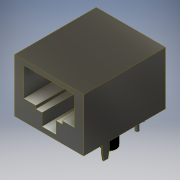
# Autodesk Inventor part: RJE051AA1310
Saved by Autodesk Inventor 2016 (Build 200138000, 138)
## iProperties
Created: 2016-08-10
Part Number: RJE051AA1310
Material: Generic
Document SubType Name: Modeling
Designer: jfixelle
Density: 1 g/cm^3
Appearance: Silver
Author: jfixelle
Autodesk Inventor part; units mm, degrees
ref_plane "YZ Plane" through (0, 0, 0) normal (1, 0, 0) x (0, 1, 0)
ref_plane "XZ Plane" through (0, 0, 0) normal (0, 1, 0) x (-1, 0, 0)
ref_plane "XY Plane" through (0, 0, 0) normal (0, 0, 1) x (1, 0, 0)
sketch "Sketch1" plane through (0, 0, 0) normal (0, 1, 0) x (-1, 0, 0)
  line L0 (7.95, 14.5) -> (-7.95, 14.5)
  line L1 (-7.95, 14.5) -> (-7.95, -4.3)
  line L2 (-7.95, -4.3) -> (7.95, -4.3)
  line L3 (7.95, -4.3) -> (7.95, 14.5)
  point P0 (0, 0)
  dimension "d0" = 18.8
  dimension "d1" = 15.9
  dimension "d2" = 7.95
  dimension "d5" = 14.5
  constraints: 8 end point, 2 parallel, 1 horizontal, 1 perpendicular
  measures "d0" distance of L2.end L0.start
  measures "d1" distance of L1.end L2.end
  measures "d2" distance from line of point (0, 0) L3
  measures "d5" distance from line of point (0, 0) L0
extrude "Extrusion1" add sketch "Sketch1" along normal blind 12.25
sketch "Sketch2" plane through (-7.95, 0, 14.5) normal (0, 0, 1) x (1, 0, 0)
  line L0 (2.12, 11.155) -> (13.78, 11.155)
  line L1 (13.78, 11.155) -> (13.78, 4.555)
  line L2 (13.78, 4.555) -> (2.12, 4.555)
  line L3 (2.12, 4.555) -> (2.12, 11.155)
  line L4 (4.9, 4.555) -> (11, 4.555)
  line L5 (11, 4.555) -> (11, 3.865)
  line L6 (11, 3.865) -> (4.9, 3.865)
  line L7 (4.9, 3.865) -> (4.9, 4.555)
  line L8 (6.325, 3.865) -> (9.575, 3.865)
  line L9 (9.575, 3.865) -> (9.575, 1.095)
  line L10 (9.575, 1.095) -> (6.325, 1.095)
  line L11 (6.325, 1.095) -> (6.325, 3.865)
  line L12 (0, 12.25) -> (15.9, 12.25) projected
  point P0 (7.95, 0)
  dimension "d6" = 11.66
  dimension "d7" = 5.83
  dimension "d8" = 6.1
  dimension "d9" = 3.05
  dimension "d10" = 3.25
  dimension "d11" = 1.625
  dimension "d12" = 7.29
  dimension "d13" = 2.77
  dimension "d14" = 6.6
  dimension "d16" = 1.095
  constraints: 24 end point, 6 parallel, 3 horizontal, 3 perpendicular, 2 point on line
  measures "d6" distance of L0.start L0.end
  measures "d7" distance from line of point (7.95, 0) L1
  measures "d8" distance of L5.end L6.end
  measures "d9" distance from line of point (7.95, 0) L5
  measures "d10" distance of L9.end L10.end
  measures "d11" distance from line of point (7.95, 0) L9
  measures "d12" distance between parallel lines of L6 L0
  measures "d13" distance between parallel lines of L10 L6
  measures "d14" distance between parallel lines of L2 L0
  measures "d16" distance between parallel lines of L12 L0
extrude "Extrusion2" cut sketch "Sketch2" against normal blind 12.32
sketch "Sketch3" plane through (7.95, 0, 14.5) normal (1, 0, 0) x (0, 0, -1)
  line L0 (4.3, 0) -> (5.9, 0)
  line L1 (5.9, 0) -> (5.9, -3.3)
  line L2 (5.9, -3.3) -> (4.3, -3.3)
  line L3 (4.3, -3.3) -> (4.3, 0)
  line L4 (0, 0) -> (0, 12.25) projected
  line L5 (4.3, -1.65) -> (4.5909, -3.3)
  line L6 (5.6091, -3.3) -> (5.9, -1.65)
  line L7 (0, 0) -> (18.8, 0) projected
  point P0 (14.5, 0)
  dimension "d19" = 3.3
  dimension "d20" = 1.6
  dimension "d21" = 4.3
  dimension "d22" = 10
  dimension "d23" = 10
  dimension "d24" = 1.65
  dimension "d25" = 0
  constraints: 12 end point, 2 midpoint, 2 parallel, 2 point on line, 1 horizontal, 1 perpendicular
  measures "d19" distance of L0.end L1.end
  measures "d20" distance of L1.end L2.end
  measures "d21" distance between parallel lines of L4 L3
  measures "d22" angle of L1 L6
  measures "d23" angle of L3 L5
  measures "d24" distance from line of L0 L5.start
  measures "d25" distance between parallel lines of L0 L7
extrude "Extrusion3" add sketch "Sketch3" against normal blind 0.3 contours L0 L1 L6 L2 L5 L3
mirror "Mirror1" about plane through (0, 0, 0) normal (1, 0, 0) of "Extrusion3"
sketch "Sketch4" plane through (0, 0, 0) normal (0, -1, 0) x (1, 0, 0)
  circle A0 centre (5.715, 6.35) radius 1.6
  line L0 (-7.95, 14.5) -> (7.95, 14.5) projected
  point P0 (0, 0)
  dimension "d28" = 3.2
  dimension "d29" = 8.15
  dimension "d30" = 5.715
  constraints: 1 centre point
  measures "d28" diameter of A0
  measures "d29" distance from line of L0 A0.centre
  measures "d30" horizontal distance of point (0, 0) A0.centre
extrude "Extrusion4" add sketch "Sketch4" along normal blind 3.25
chamfer "Chamfer1" distance 0.25 angle 45 1 edges at (4.115, -3.25, 6.35)
sketch "Sketch5" plane through (5.715, -3.25, 6.35) normal (0, -1, 0) x (1, 0, 0)
  line L0 (0.7635, 1.8366) -> (0.2859, 1.8366)
  line L1 (0.2859, 1.8366) -> (0.2859, -1.8337)
  line L2 (0.2859, -1.8337) -> (0.7635, -1.8337)
  line L3 (0.7635, -1.8337) -> (0.7635, 1.8366)
  point P0 (-5.715, -6.35)
  constraints: 8 end point, 2 parallel, 1 horizontal, 1 perpendicular
extrude "Extrusion5" cut sketch "Sketch5" against normal blind 3.25
fillet "Fillet1" radius 0.25 1 edges at (6.0009, 0, 6.35)
fillet "Fillet2" radius 0.2 1 edges at (6.4785, 0, 6.35)
mirror "Mirror2" about plane through (0, 0, 0) normal (1, 0, 0) of "Extrusion4", "Chamfer1", "Extrusion5", "Fillet1", "Fillet2"
sketch "Sketch6" plane through (0, 0, 0) normal (0, -1, 0) x (1, 0, 0)
  line L0 (3.8973, 0) -> (-6.9227, 0) construction
  line L1 (4.2984, -2.54) -> (-6.5216, -2.54) construction
  circle A0 centre (0.635, 0) radius 0.4
  circle A1 centre (-0.635, -2.54) radius 0.4
  circle A2 centre (-3.175, -2.54) radius 0.4
  circle A3 centre (-5.715, -2.54) radius 0.4
  circle A4 centre (1.905, -2.54) radius 0.4
  circle A5 centre (-0.635, -2.54) radius 0.4
  circle A6 centre (-3.175, -2.54) radius 0.4
  circle A7 centre (4.445, -2.54) radius 0.4
  circle A8 centre (1.905, -2.54) radius 0.4
  circle A9 centre (-0.635, -2.54) radius 0.4
  circle A10 centre (-1.905, 0) radius 0.4
  circle A11 centre (-4.445, 0) radius 0.4
  circle A12 centre (3.175, 0) radius 0.4
  circle A13 centre (0.635, 0) radius 0.4
  circle A14 centre (-1.905, 0) radius 0.4
  circle A15 centre (5.715, 0) radius 0.4
  circle A16 centre (3.175, 0) radius 0.4
  circle A17 centre (0.635, 0) radius 0.4
  point P0 (0, 0)
  dimension "d40" = 2.54
  dimension "d41" = 0
  dimension "d45" = 0.8
  dimension "d46" = 0.8
  dimension "d49" = 2.54
  dimension "d52" = 2.54
  dimension "d57" = 2.54
  dimension "d60" = 2.54
  dimension "d63" = 0.635
  dimension "d64" = 0.635
  constraints: 18 centre point, 6 horizontal, 4 end point, 2 point on line, 32 other
  measures "d40" distance between parallel lines of L1 L0
  measures "d41" distance from line of point (0, 0) L0
  measures "d45" diameter of A1
  measures "d46" diameter of A0
  measures "d49" distance of A1.centre A2.centre
  measures "d52" distance of A1.centre A4.centre
  measures "d57" distance of A0.centre A10.centre
  measures "d60" distance of A0.centre A12.centre
  measures "d63" distance of point (0, 0) A0.centre
  measures "d64" horizontal distance of point (0, 0) A9.centre
extrude "Extrusion6" add sketch "Sketch6" along normal blind 3.25
body "Solid1"
